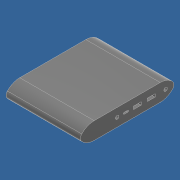
# Autodesk Inventor part: batter_krisdonia
Saved by Autodesk Inventor 2022.4 (Build 264492000, 492)
## iProperties
Created: 2023-07-26
Part Number: batter_krisdonia
Material: 一般
Document SubType Name: Modeling
Designer: 8326d
Density: 1 g/cm^3
Appearance: 滑らか - 黒
Author: 8326d
Autodesk Inventor part; units mm, degrees
ref_plane "YZ Plane" through (0, 0, 0) normal (1, 0, 0) x (0, 1, 0)
ref_plane "XZ Plane" through (0, 0, 0) normal (0, 1, 0) x (-1, 0, 0)
ref_plane "XY Plane" through (0, 0, 0) normal (0, 0, 1) x (1, 0, 0)
sketch "スケッチ1" plane through (0, 0, 0) normal (1, 0, 0) x (0, 1, 0)
  line L0 (-14.5, 81) -> (14.5, 81)
  line L1 (14.5, 81) -> (14.5, -81)
  line L2 (14.5, -81) -> (-14.5, -81)
  line L3 (-14.5, -81) -> (-14.5, 81)
  line L4 (-14.5, 81) -> (14.5, -81) construction
  line L5 (14.5, 81) -> (-14.5, -81) construction
  arc A0 (14.5, 55.8853) -> (0, 81) centre (-14.5, 55.8853) ccw
  arc A1 (0, 81) -> (-14.5, 55.8853) centre (14.5, 55.8853) ccw
  arc A2 (0, -81) -> (14.5, -55.8853) centre (-14.5, -55.8853) ccw
  arc A3 (-14.5, -55.8853) -> (0, -81) centre (14.5, -55.8853) ccw
  point P0 (0, 0)
  dimension "d0" = 29
  dimension "d1" = 162
  constraints: 12 end point, 8 point on circle, 4 centre point, 4 midpoint, 4 point on line, 2 coincident, 2 parallel, 2 tangent, 1 horizontal, 1 perpendicular
  measures "d0" distance of L1.end L2.end
  measures "d1" distance of L0.end L1.end
extrude "押し出し1" add sketch "スケッチ1" along normal mid plane 126 contours A0 L1 A2 A3 L3 A1
fillet "フィレット1" radius 8 2 edges at (0, 0, 81) (0, 0, -81)
sketch "スケッチ2" plane through (63, 0, 0) normal (1, 0, 0) x (0, 0, -1)
  arc A0 (-76.8626, 5.5238) -> (-76.8626, -5.5238) centre (-71.0757, 0) ccw projected
  arc A1 (76.8626, -5.5238) -> (76.8626, 5.5238) centre (71.0757, 0) ccw projected
  line L0 (-71.0757, 0) -> (71.0757, 0) construction
  circle A2 centre (65.0757, 0) radius 3
  circle A3 centre (-16.9243, 0) radius 3
  line L1 (34.0757, 2.5) -> (47.0757, 2.5)
  line L2 (47.0757, 2.5) -> (47.0757, -2.5)
  line L3 (47.0757, -2.5) -> (34.0757, -2.5)
  line L4 (34.0757, -2.5) -> (34.0757, 2.5)
  line L5 (34.0757, 2.5) -> (47.0757, -2.5) construction
  line L6 (47.0757, 2.5) -> (34.0757, -2.5) construction
  line L7 (10.5757, 2.5) -> (23.5757, 2.5)
  line L8 (23.5757, 2.5) -> (23.5757, -2.5)
  line L9 (23.5757, -2.5) -> (10.5757, -2.5)
  line L10 (10.5757, -2.5) -> (10.5757, 2.5)
  line L11 (10.5757, 2.5) -> (23.5757, -2.5) construction
  line L12 (23.5757, 2.5) -> (10.5757, -2.5) construction
  line L13 (-4.9243, 0) -> (1.0757, 0) construction
  line L14 (-4.9243, -1.5) -> (1.0757, -1.5)
  line L15 (1.0757, 1.5) -> (-4.9243, 1.5)
  arc A4 (-4.9243, 1.5) -> (-4.9243, -1.5) centre (-4.9243, 0) ccw
  arc A5 (1.0757, -1.5) -> (1.0757, 1.5) centre (1.0757, 0) ccw
  point P0 (0, 0)
  point P1 (40.5757, 0)
  point P2 (17.0757, 0)
  point P3 (40.5757, 0)
  point P4 (17.0757, 0)
  point P5 (-1.9243, 0)
  point P6 (0, 0)
  dimension "d5" = 6
  dimension "d6" = 6
  dimension "d7" = 6
  dimension "d8" = 88
  dimension "d9" = 13
  dimension "d10" = 5
  dimension "d11" = 13
  dimension "d12" = 5
  dimension "d13" = 24.5
  dimension "d14" = 48
  dimension "d15" = 73
  dimension "d16" = 1.5
  dimension "d18" = 6
  constraints: 32 end point, 7 midpoint, 5 parallel, 4 centre point, 4 point on circle, 4 tangent, 2 horizontal, 2 perpendicular, 10 other
  measures "d5" diameter of A2
  measures "d6" diameter of A3
  measures "d7" distance of A1.centre A2.centre
  measures "d8" distance of A1.centre A3.centre
  measures "d9" distance of L2.end L3.end
  measures "d10" distance of L1.end L2.end
  measures "d11" distance of L8.end L9.end
  measures "d12" distance of L7.end L8.end
  measures "d13" distance of A2.centre point (40.576, 0)
  measures "d14" distance of A2.centre point (17.076, 0)
  measures "d15" distance of A1.centre point (-1.924, 0)
  measures "d16" radius of A4
  measures "d18" distance of L13.start L13.end
extrude "押し出し2" cut sketch "スケッチ2" against normal blind 5
